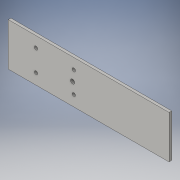
# Autodesk Inventor part: VersaPlate
Saved by Autodesk Inventor 2016 (Build 200138000, 138)
## iProperties
Created: 2016-02-15
Part Number: VersaPlate
Material: Generic
Document SubType Name: Modeling
Designer: Mentor1102
Density: 1 g/cm^3
Appearance: Default
Author: Mentor1102
Autodesk Inventor part; units mm, degrees
ref_plane "YZ Plane" through (0, 0, 0) normal (1, 0, 0) x (0, 1, 0)
ref_plane "XZ Plane" through (0, 0, 0) normal (0, 1, 0) x (-1, 0, 0)
ref_plane "XY Plane" through (0, 0, 0) normal (0, 0, 1) x (1, 0, 0)
sketch "Sketch1" plane through (0, 0, 0) normal (0, 0, 1) x (1, 0, 0)
  circle A0 centre (26.7, 1.3) radius 2.0193
  circle A1 centre (25.2, 14) radius 2.5
  circle A2 centre (26.7, 26.7) radius 2.0193
  circle A3 centre (-18.1314, 26.7) radius 2.0193
  circle A4 centre (-18.1314, 1.3) radius 2.0193
  line L0 (25.2, 14) -> (139.5, 14) construction
  line L1 (139.5, 14) -> (139.5, 39.4)
  line L2 (139.5, 14) -> (139.5, -11.4)
  line L3 (139.5, -11.4) -> (-51, -11.4)
  line L4 (-51, -11.4) -> (-51, 39.4)
  line L5 (-51, 39.4) -> (139.5, 39.4)
  point P0 (0, 0)
  dimension "d0" = 114.3
  dimension "d1" = 25.4
  dimension "d2" = 25.4
  dimension "d3" = 190.5
  dimension "d6" = 44.8314
  constraints: 12 end point, 5 centre point, 2 perpendicular, 2 vertical, 1 horizontal, 1 parallel
  measures "d0" distance of L0.start L0.end
  measures "d1" distance of L0.end L1.end
  measures "d2" distance of L0.end L2.end
  measures "d3" distance of L2.end L3.end
  measures "d6" distance of A3.centre A2.centre
extrude "Extrusion1" add sketch "Sketch1" along normal blind 3.175
body "Solid1"
